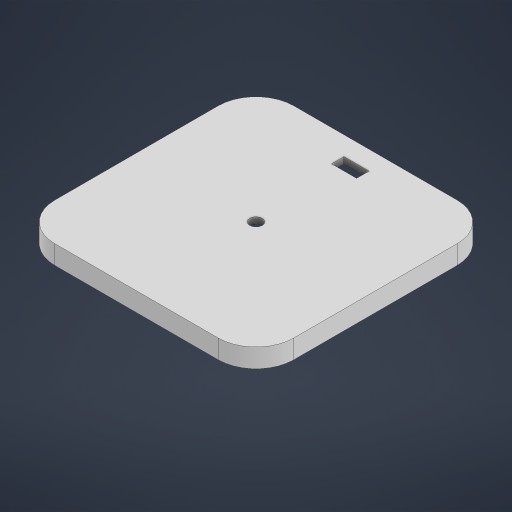
# Autodesk Inventor part: top
Saved by Autodesk Inventor 2024 (Build 280153000, 153)
## iProperties
Created: 2023-06-18
Part Number: top
Material: 일반
Document SubType Name: Modeling
Designer: 6gioc
Density: 1 g/cm^3
Appearance: 기본값
Author: 6gioc
## iProperties of the stored document top_3D 인쇄.ipt
Created: 2023-06-20
Part Number: top_3D 인쇄
Material: 일반
Document SubType Name: Modeling
Designer: 6gioc
Density: 1 g/cm^3
Appearance: 기본값
Author: 6gioc
Autodesk Inventor part; units mm, degrees
ref_plane "YZ Plane" through (0, 0, 0) normal (1, 0, 0) x (0, 1, 0)
ref_plane "XZ Plane" through (0, 0, 0) normal (0, 1, 0) x (-1, 0, 0)
ref_plane "XY Plane" through (0, 0, 0) normal (0, 0, 1) x (1, 0, 0)
sketch "스케치1" plane through (0, 0, 0) normal (0, 1, 0) x (-1, 0, 0)
  line L0 (30, 0) -> (160, 0)
  line L1 (190, -30) -> (190, -160)
  line L2 (160, -190) -> (30, -190)
  line L3 (0, -160) -> (0, -30)
  arc A0 (190, -30) -> (160, 0) centre (160, -30) ccw
  arc A1 (160, -190) -> (190, -160) centre (160, -160) ccw
  arc A2 (0, -160) -> (30, -190) centre (30, -160) ccw
  arc A3 (30, 0) -> (0, -30) centre (30, -30) ccw
  point P0 (0, 0)
  point P1 (190, -190)
  point P2 (190, 0)
  point P3 (0, -190)
  dimension "d0" = 190
  dimension "d1" = 190
  dimension "d2" = 30
  constraints: 8 end point, 8 point on circle, 8 point on line, 8 tangent, 4 centre point, 3 equal radius, 2 parallel, 1 horizontal, 1 perpendicular
  measures "d0" distance of point (190, -190) point (0, -190)
  measures "d1" distance of point (190, 0) point (190, -190)
  measures "d2" radius of A0
extrude "돌출1" add sketch "스케치1" along normal blind 15
shell "쉘1" thickness 5 removed faces 1 at (-106.6667, 0, -116.6667)
sketch "스케치3" plane through (0, 15, 0) normal (0, 1, 0) x (1, 0, 0)
  circle A0 centre (-95, 95) radius 5
  line L0 (-190, 160) -> (-190, 30) projected
  line L1 (-160, 0) -> (-30, 0) projected
  line L2 (-105, 175) -> (-85, 175)
  line L3 (-85, 175) -> (-85, 165)
  line L4 (-85, 165) -> (-105, 165)
  line L5 (-105, 165) -> (-105, 175)
  line L6 (-30, 190) -> (-160, 190) projected
  point P0 (0, 0)
  point P1 (-105, 170)
  dimension "d12" = 10
  dimension "d13" = 95
  dimension "d14" = 95
  dimension "d15" = 20
  dimension "d16" = 10
  dimension "d17" = 85
  dimension "d18" = 15
  constraints: 8 end point, 2 parallel, 1 centre point, 1 horizontal, 1 midpoint, 1 perpendicular
  measures "d12" diameter of A0
  measures "d13" distance from line of A0.centre L0
  measures "d14" distance from line of L1 A0.centre
  measures "d15" distance of L3.end L4.end
  measures "d16" distance of L2.end L3.end
  measures "d17" distance from line of L0 point (-105, 170)
  measures "d18" distance between parallel lines of L6 L2
extrude "돌출3" cut sketch "스케치3" against normal blind 10
sketch "스케치4" plane through (-160, 10, -185) normal (0, -1, 0) x (1, 0, 0)
  circle A0 centre (65, 90) radius 22
  circle A1 centre (65, 90) radius 5 projected
  line L0 (71, 130) -> (113, 130)
  line L1 (113, 130) -> (113, 128)
  line L2 (113, 128) -> (71, 128)
  line L3 (71, 128) -> (71, 130)
  line L4 (130, 0) -> (0, 0) projected
  line L5 (155, 155) -> (155, 25) projected
  line L6 (0, 180) -> (130, 180) projected
  point P0 (160, 185)
  point P1 (113, 129)
  dimension "d21" = 44
  dimension "d22" = 42
  dimension "d23" = 2
  dimension "d25" = 42
  dimension "d28" = 50
  constraints: 8 end point, 2 parallel, 1 centre point, 1 concentric, 1 horizontal, 1 midpoint, 1 perpendicular
  measures "d21" diameter of A0
  measures "d22" distance of L1.end L2.end
  measures "d23" distance of L0.end L1.end
  measures "d25" distance from line of L5 point (113, 129)
  measures "d28" distance between parallel lines of L6 L0
extrude "돌출4" add sketch "스케치4" along normal blind 42 contours L0 L1 L2 L3
sketch "스케치5" plane through (-47, 10, -57) normal (0, 0, -1) x (-1, 0, 0)
  circle A0 centre (5.5, -36.5) radius 1.5
  circle A1 centre (36.5, -36.5) radius 1.5
  circle A2 centre (36.5, -5.5) radius 1.5
  circle A3 centre (5.5, -5.5) radius 1.5
  line L0 (42, 0) -> (42, -42) projected
  line L1 (0, 0) -> (0, -42) projected
  line L2 (42, -42) -> (0, -42) projected
  circle A4 centre (21, -21) radius 11
  point P0 (-47, -10)
  dimension "d29" = 3
  dimension "d30" = 3
  dimension "d31" = 3
  dimension "d32" = 3
  dimension "d33" = 31
  dimension "d34" = 31
  dimension "d35" = 31
  dimension "d36" = 31
  dimension "d37" = 31
  dimension "d38" = 31
  dimension "d39" = 42
  dimension "d40" = 5.5
  dimension "d41" = 5.5
  dimension "d44" = 22
  dimension "d45" = 21
  dimension "d46" = 21
  constraints: 5 centre point
  measures "d29" diameter of A0
  measures "d30" diameter of A1
  measures "d31" diameter of A2
  measures "d32" diameter of A3
  measures "d33" distance of A2.centre A3.centre
  measures "d34" distance of A1.centre A2.centre
  measures "d35" distance of A0.centre A1.centre
  measures "d36" distance of A3.centre A0.centre
  measures "d37" horizontal distance of A2.centre A0.centre
  measures "d38" horizontal distance of A1.centre A3.centre
  measures "d39" distance between parallel lines of L0 L1
  measures "d40" distance from line of L1 A0.centre
  measures "d41" distance from line of L2 A0.centre
  measures "d44" diameter of A4
  measures "d45" distance from line of L1 A4.centre
  measures "d46" distance from line of L2 A4.centre
extrude "돌출5" cut sketch "스케치5" against normal blind 42
